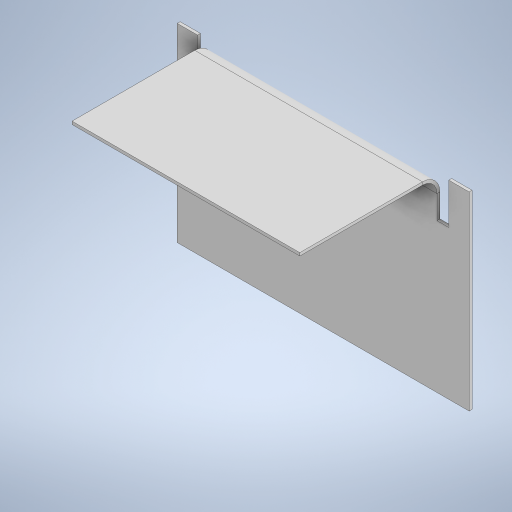
# Autodesk Inventor part: Ex 1
Saved by Autodesk Inventor 2023.2 (Build 272271000, 271)
## iProperties
Created: 2022-12-21
Part Number: Ex 1
Material: Generic
Document SubType Name: Sheet Metal
Designer: Felipe Coquito
Density: 1 g/cm^3
Sheet Metal Rule: Default_mm
Appearance: Default
Author: Felipe Coquito
Autodesk Inventor part; units mm, degrees
ref_plane "YZ Plane" through (0, 0, 0) normal (1, 0, 0) x (0, 1, 0)
ref_plane "XZ Plane" through (0, 0, 0) normal (0, 1, 0) x (-1, 0, 0)
ref_plane "XY Plane" through (0, 0, 0) normal (0, 0, 1) x (1, 0, 0)
sketch "Sketch1" plane through (0, 0, 0) normal (0, 0, 1) x (1, 0, 0)
  line L0 (-50, 32.5) -> (50, 32.5)
  line L1 (50, 32.5) -> (50, -32.5)
  line L2 (50, -32.5) -> (-50, -32.5)
  line L3 (-50, -32.5) -> (-50, 32.5)
  line L4 (-50, 32.5) -> (50, -32.5) construction
  line L5 (50, 32.5) -> (-50, -32.5) construction
  point P0 (0, 0)
  dimension "d0" = 100
  dimension "d1" = 65
  measures "d0" distance of L1.end L2.end
  measures "d1" distance of L0.end L1.end
extrude "Plate1" add sketch "Sketch1" along normal blind 1
sketch "Sketch3" plane through (-50, 31.5, 0) normal (0, 1, 0) x (-1, 0, 0)
  line L0 (-89, 0) -> (-11, 0)
  line L1 (-11, 0) -> (-11, 48)
  line L2 (-11, 48) -> (-89, 48)
  line L3 (-89, 48) -> (-89, 0)
  constraints: 8 end point
edge flange "Flange1" height 48 angle 90 thickness 1 bend radius 5 thickness toward (0, 1, 0) relief straight relief width 4 relief depth 8 edges at (0, 32.5, 1) wall of the first edge with corners at (39, 31.5, 0) (-39, 31.5, 0) (-39, 31.5, 48) (39, 31.5, 48)
bend "Bend1"
corner "Corner1"
equation "\"d2\" = Thickness"
equation "\"d6\" = TransitionRadius"
equation "\"d12\" = CornerReliefSize"
equation "\"d13\" = GapSize"
equation "\"d14\" = JacobiRadiusSize"
equation "\"GapSize\" = Thickness"
equation "\"BendRadius\" = Thickness"
equation "\"MinimumRemnant\" = 2 * Thickness"
equation "\"BendReliefDepth\" = 0.5 * Thickness"
equation "\"BendReliefWidth\" = Thickness"
equation "\"CornerReliefSize\" = 4 * Thickness"
equation "\"JacobiRadiusSize\" = BendRadius"
equation "\"TransitionRadius\" = BendRadius"
equation "\"Thickness\" = 1"
body "Solid1"
